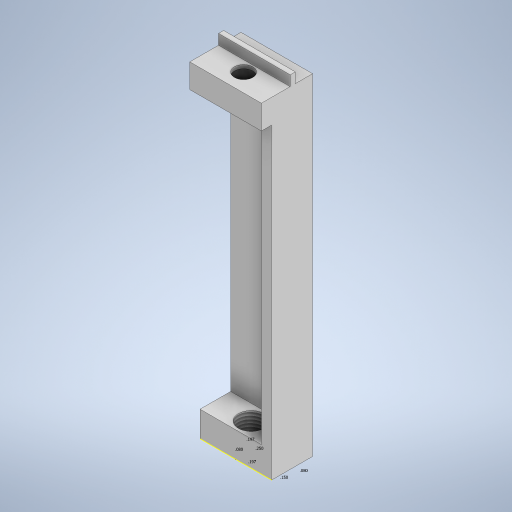
# Autodesk Inventor part: IDA12toPolarisAdapter
Saved by Autodesk Inventor 2024.2 (Build 282272000, 272)
## iProperties
Created: 2024-12-03
Part Number: IDA12toPolarisAdapter
Material: Generic
Document SubType Name: Modeling
Designer: monolithic
Density: 1 g/cm^3
Appearance: Default
Author: monolithic
Autodesk Inventor part; units mm, degrees
ref_plane "YZ Plane" through (0, 0, 0) normal (1, 0, 0) x (0, 1, 0)
ref_plane "XZ Plane" through (0, 0, 0) normal (0, 1, 0) x (-1, 0, 0)
ref_plane "XY Plane" through (0, 0, 0) normal (0, 0, 1) x (1, 0, 0)
sketch "Sketch1" plane through (0, 0, 0) normal (0, 1, 0) x (-1, 0, 0)
  line L0 (0, 0) -> (-17.78, 0)
  line L1 (-17.78, 0) -> (-17.78, -10.16)
  line L2 (-17.78, -10.16) -> (0, -10.16)
  line L3 (0, -10.16) -> (0, 0)
  dimension "d0" = 17.78
  dimension "d1" = 10.16
  constraints: 8 end point, 2 parallel, 1 horizontal, 1 perpendicular
  measures "d0" distance of L1.end L2.end
  measures "d1" distance of L0.end L1.end
extrude "Extrusion1" add sketch "Sketch1" along normal blind 82.296
sketch "Sketch2" plane through (0, 0, 0) normal (0, -1, 0) x (1, 0, 0)
  line L0 (0, 0) -> (0, -5.08)
  line L1 (0, -10.16) -> (0, 0) projected
  line L2 (0, 0) -> (17.78, 0) projected
  line L3 (8.89, 0) -> (8.89, -3.81)
  circle A0 centre (8.89, -3.81) radius 3.175
  line L4 (8.89, -3.81) -> (11.8809, -3.81)
  line L5 (8.89, -3.81) -> (3.8862, -3.81)
  line L6 (8.89, -3.81) -> (13.8938, -3.81)
  circle A1 centre (13.8938, -3.81) radius 1.016
  circle A2 centre (3.8862, -3.81) radius 1.016
  dimension "d5" = 6.35
  dimension "d6" = 5.0038
  dimension "d7" = 5.0038
  dimension "d8" = 2.032
  dimension "d9" = 2.032
  dimension "d20" = 3.81
  constraints: 10 end point, 3 centre point, 3 coincident, 3 horizontal, 2 midpoint, 1 vertical
  measures "d5" diameter of A0
  measures "d6" distance of L4.start L5.end
  measures "d7" distance of L4.start L6.end
  measures "d8" diameter of A2
  measures "d9" diameter of A1
  measures "d20" distance of L3.start L3.end
extrude "Extrusion2" cut sketch "Sketch2" against normal blind 50.8 contours A0 L6 L4 L3 | L3 L5 A0 | L4 L6 A0 L5
sketch "Sketch3" plane through (0, 0, 0) normal (0, 0, 1) x (1, 0, 0)
  line L0 (0, 0) -> (0, 82.296) projected
  line L1 (0, 0) -> (0, 6.35)
  line L2 (0, 6.35) -> (15.24, 6.35)
  line L3 (15.24, 6.35) -> (-24.1406, 6.35)
  line L4 (-24.1406, 6.35) -> (-24.1406, 76.3224)
  line L5 (-24.1406, 76.3224) -> (15.24, 76.3224)
  line L6 (15.24, 76.3224) -> (15.24, 6.35)
  point P0 (0, 76.3224)
  dimension "d12" = 6.35
  dimension "d13" = 15.24
  constraints: 12 end point, 2 parallel, 2 perpendicular, 1 horizontal, 1 point on line
  measures "d12" distance of L0.start L1.end
  measures "d13" distance of L1.end L2.end
extrude "Extrusion3" cut sketch "Sketch3" against normal blind 7.62 contours L0 L5 L6 L2
extrude "Extrusion4" cut sketch "Sketch2" against normal blind 4.445 contours A1 | A2
thread "Thread1" size "8-32 UNC" class "2B" standard "ANSI Unified Screw Threads" length 9.896
sketch "Sketch4" plane through (0, 82.296, 0) normal (0, 1, 0) x (1, 0, 0)
  circle A0 centre (8.89, 3.81) radius 3.175 projected
  line L0 (8.89, 0) -> (8.89, 3.81) projected
  circle A1 centre (8.89, 3.81) radius 2.286
  line L1 (8.89, 3.81) -> (8.89, 1.9304)
  circle A2 centre (8.89, 1.9304) radius 2.286
  point P0 (0, 0)
  dimension "d21" = 4.572
  dimension "d28" = 1.8796
  dimension "d29" = 4.572
  constraints: 2 centre point, 2 coincident, 2 end point, 1 point on line
  measures "d21" diameter of A1
  measures "d28" distance of L1.start L1.end
  measures "d29" diameter of A2
sketch "Sketch5" plane through (0, 82.296, 0) normal (0, 1, 0) x (1, 0, 0)
  circle A0 centre (8.89, 3.81) radius 2.286 projected
  line L0 (8.89, 3.81) -> (8.89, 6.477)
  line L1 (8.89, 6.477) -> (0, 6.477)
  line L2 (0, 10.16) -> (0, 0) projected
  line L3 (8.89, 6.477) -> (17.78, 6.477)
  line L4 (17.78, 0) -> (17.78, 10.16) projected
  line L5 (17.78, 6.477) -> (17.78, 7.747)
  line L6 (17.78, 7.747) -> (0, 7.747)
  line L7 (0, 6.477) -> (0, 7.747)
  line L8 (8.89, 3.81) -> (8.89, 1.9304)
  line L9 (8.89, 6.477) -> (8.89, 4.5974)
  line L10 (8.89, 4.5974) -> (0, 4.5974)
  line L11 (8.89, 4.5974) -> (17.78, 4.5974)
  line L12 (17.78, 5.8674) -> (0, 5.8674)
  line L13 (17.78, 4.5974) -> (17.78, 5.8674)
  line L14 (0, 4.5974) -> (0, 5.8674)
  point P0 (0, 5.8674)
  point P1 (0, 4.5974)
  dimension "d24" = 2.667
  dimension "d25" = 1.27
  dimension "d35" = 1.8796
  dimension "d36" = 1.8796
  dimension "d37" = 1.27
  constraints: 26 end point, 5 point on line, 4 horizontal, 2 perpendicular, 2 vertical, 1 collinear, 1 parallel
  measures "d24" distance of L0.start L0.end
  measures "d25" distance of L3.end L5.end
  measures "d35" distance of L0.start L8.end
  measures "d36" distance of L0.end L9.end
  measures "d37" distance of L11.end L12.start
sketch "Sketch6" plane through (0, 82.296, 0) normal (0, 1, 0) x (1, 0, 0)
  line L0 (0, 0) -> (17.78, 0) projected
  line L1 (0, 0) -> (17.78, 0)
  line L2 (17.78, 0) -> (17.78, -2.54)
  line L3 (17.78, -2.54) -> (0, -2.54)
  line L4 (0, -2.54) -> (0, 0)
  dimension "d30" = 2.54
  constraints: 8 end point, 3 perpendicular, 1 collinear
  measures "d30" distance of L0.end L2.end
extrude "Extrusion7" add sketch "Sketch6" against normal blind 5.9736
extrude "Extrusion8" cut sketch "Sketch4" against normal blind 25.4 contours A2 A1 L0 A0 | A0 A2 | A0 L0 A1 A2 | A2 A1 picked at (9.0633, 2.4414)
extrude "Extrusion9" add sketch "Sketch5" along normal blind 2.54 contours L11 L0 L12 A0 | A0 L12 L4 L11 | L10 L2 L12 A0 | A0 L12 L0 L10
sketch "Sketch8" plane through (0, 76.3224, -7.62) normal (0, -1, 0) x (1, 0, 0)
  circle A0 centre (8.89, 5.6896) radius 2.286 projected
  circle A1 centre (8.89, 5.6896) radius 2.286 projected
  circle A2 centre (8.89, 5.6896) radius 3.81
  point P0 (0, 7.62)
  point P1 (10.1145, 7.62)
  point P2 (7.6655, 7.62)
  dimension "d41" = 7.62
  constraints: 1 centre point, 1 coincident
  measures "d41" diameter of A2
extrude "Extrusion10" cut sketch "Sketch8" against normal blind 5.08
body "Solid1"
